Autodesk Inventor part; units mm, degrees
(part 2 of 2)
  spline S143 degree 2 poles (-142.6782, 115.4666) (-142.2668, 115.4666) (-141.7097, 116.001) (-141.7097, 116.3572) knots 0 0 0 1 2 2 2
  spline S144 degree 2 poles (-141.7097, 116.3572) (-141.7097, 116.5807) (-141.9494, 116.9694) (-142.3769, 117.1832) (-142.6587, 117.1832) knots 0 0 0 1 2 3 3 3
  spline S145 degree 2 poles (-142.6587, 117.1832) (-143.0927, 117.1832) (-143.6077, 116.6649) (-143.6077, 116.3216) knots 0 0 0 1 2 2 2
  spline S146 degree 2 poles (-143.6077, 116.3216) (-143.6077, 115.9848) (-143.0636, 115.4666) (-142.6782, 115.4666) knots 0 0 0 1 2 2 2
  spline S147 degree 2 poles (-142.662, 113.75) (-142.3316, 113.75) (-141.9008, 114.1386) (-141.9008, 114.4074) knots 0 0 0 1 2 2 2
  spline S148 degree 2 poles (-141.9008, 114.4074) (-141.9008, 114.673) (-142.364, 115.1038) (-142.6749, 115.1038) knots 0 0 0 1 2 2 2
  spline S149 degree 2 poles (-142.6749, 115.1038) (-142.8725, 115.1038) (-143.2255, 114.9095) (-143.4231, 114.5694) (-143.4231, 114.3977) knots 0 0 0 1 2 3 3 3
  spline S150 degree 2 poles (-143.4231, 114.3977) (-143.4231, 114.1581) (-143.0312, 113.75) (-142.662, 113.75) knots 0 0 0 1 2 2 2
  spline S151 degree 2 poles (-144.3786, 115.4633) (-144.3786, 114.673) (-144.7186, 113.8083) (-145.3405, 113.3613) (-145.7227, 113.3613) knots 0 0 0 1 2 3 3 3
  spline S152 degree 2 poles (-145.7227, 113.3613) (-146.1114, 113.3613) (-146.7462, 113.8115) (-147.1122, 114.7087) (-147.1122, 115.4633) knots 0 0 0 1 2 3 3 3
  spline S153 degree 2 poles (-147.1122, 115.4633) (-147.1122, 116.2147) (-146.7494, 117.1087) (-146.1114, 117.5621) (-145.7227, 117.5621) knots 0 0 0 1 2 3 3 3
  spline S154 degree 2 poles (-145.7227, 117.5621) (-145.3405, 117.5621) (-144.7251, 117.1216) (-144.3786, 116.2504) (-144.3786, 115.4633) knots 0 0 0 1 2 3 3 3
  spline S155 degree 2 poles (-144.7575, 115.4698) (-144.7575, 116.1467) (-145.0004, 116.8398) (-145.4733, 117.1993) (-145.7389, 117.1993) knots 0 0 0 1 2 3 3 3
  spline S156 degree 2 poles (-145.7389, 117.1993) (-146.0045, 117.1993) (-146.4676, 116.8496) (-146.5875, 116.4965) knots 0 0 0 1 2 2 2
  spline S157 degree 2 poles (-146.5875, 116.4965) (-146.7365, 116.0722) (-146.7365, 115.4698) knots 0 0 0 1 1 1
  spline S158 degree 2 poles (-146.7365, 115.4698) (-146.7365, 114.8674) (-146.4709, 114.0965) (-145.998, 113.7402) (-145.7389, 113.7402) knots 0 0 0 1 2 3 3 3
  spline S159 degree 2 poles (-145.7389, 113.7402) (-145.4701, 113.7402) (-145.0037, 114.0965) (-144.7575, 114.7896) (-144.7575, 115.4698) knots 0 0 0 1 2 3 3 3
  line L437 (-148.3203, 113.4617) -> (-149.1073, 113.4617)
  line L438 (-149.1073, 113.4617) -> (-149.1073, 117.4617)
  line L439 (-149.1073, 117.4617) -> (-148.7089, 117.4617)
  line L440 (-148.7089, 117.4617) -> (-148.7089, 113.8536)
  line L441 (-148.7089, 113.8536) -> (-148.0806, 113.8536)
  line L442 (-148.0806, 113.8536) -> (-148.3203, 113.4617)
  line L443 (-151.0182, 114.7119) -> (-150.6361, 114.7119)
  spline S160 degree 2 poles (-150.6361, 114.7119) (-150.6522, 114.1192) (-151.4101, 113.3613) (-151.9705, 113.3613) knots 0 0 0 1 2 2 2
  spline S161 degree 2 poles (-151.9705, 113.3613) (-152.5211, 113.3613) (-153.2045, 114.0738) (-153.2045, 114.5564) knots 0 0 0 1 2 2 2
  spline S162 degree 2 poles (-153.2045, 114.5564) (-153.2045, 114.8965) (-152.8773, 115.4925) (-152.4077, 116.001) knots 0 0 0 1 2 2 2
  line L444 (-152.4077, 116.001) -> (-151.4134, 117.0763)
  line L445 (-151.4134, 117.0763) -> (-153.2595, 117.0763)
  line L446 (-153.2595, 117.0763) -> (-153.2595, 117.4617)
  line L447 (-153.2595, 117.4617) -> (-150.5421, 117.4617)
  line L448 (-150.5421, 117.4617) -> (-152.0709, 115.8099)
  spline S163 degree 2 poles (-152.0709, 115.8099) (-152.5373, 115.3143) (-152.8158, 114.8317) (-152.8158, 114.5661) knots 0 0 0 1 2 2 2
  spline S164 degree 2 poles (-152.8158, 114.5661) (-152.8158, 114.2261) (-152.3105, 113.7402) (-151.9478, 113.7402) knots 0 0 0 1 2 2 2
  spline S165 degree 2 poles (-151.9478, 113.7402) (-151.5624, 113.7402) (-151.0539, 114.252) (-151.0182, 114.7119) knots 0 0 0 1 2 2 2
  point P0 (0, 0)
  constraints: 2 other
emboss "Emboss1" sketch "Sketch3" operation add depth 0.1 direction (0, 0, -1)
sketch "Sketch4" plane through (0, 0, 3.2) normal (0, 0, 1) x (1, 0, 0)
  line L0 (-120, -120) -> (-60, -120)
  line L1 (-60, -120) -> (-60, -80)
  line L2 (-60, -80) -> (-120, -80)
  line L3 (-120, -80) -> (-120, -120)
  line L4 (-200, -125) -> (200, -125) projected
  line L5 (-200, 125) -> (-200, -125) projected
  circle A0 centre (-143.3589, -112.9) radius 2
  line L6 (-160.8589, -102.9) -> (-155.8589, -102.9) projected
  line L7 (-158.3589, -102.9) -> (-158.3589, -106.6656) construction
  circle A1 centre (-173.3589, -112.9) radius 2
  line L8 (-200, -125) -> (200, -125) projected
  line L9 (0, -125) -> (0, -86.2229) construction
  line L10 (-200, 125) -> (-200, -125) projected
  line L11 (-200, 0) -> (-175.4594, 0) construction
  circle A2 centre (-190, 115) radius 2
  line L12 (200, 125) -> (-200, 125) projected
  circle A3 centre (-190, -115) radius 2
  circle A4 centre (190, 115) radius 2
  circle A5 centre (190, -115) radius 2
  point P0 (0, 0)
  dimension "d10" = 60
  dimension "d11" = 40
  dimension "d12" = 5
  dimension "d13" = 80
  dimension "d16" = 4
  dimension "d17" = 15
  dimension "d18" = 10
  dimension "d19" = 4
  dimension "d20" = 10
  dimension "d21" = 10
  constraints: 14 end point, 6 centre point, 4 symmetric about line, 3 midpoint, 2 horizontal, 2 parallel, 2 vertical, 1 perpendicular, 4 other
  measures "d10" distance of L2.end L1.end
  measures "d11" distance of L1.end L0.end
  measures "d12" distance between parallel lines of L0 L4
  measures "d13" distance between parallel lines of L3 L5
  measures "d16" diameter of A0
  measures "d17" horizontal distance of A0.centre L7.end
  measures "d18" distance from line of A0.centre L6
  measures "d19" diameter of A2
  measures "d20" distance from line of L12 A2.centre
  measures "d21" distance from line of L5 A2.centre
extrude "Extrusion3" cut sketch "Sketch4" against normal blind 15
equation "\"d14\" = d17"
body "Solid1"
